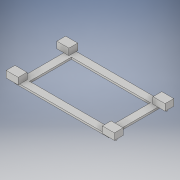
# Autodesk Inventor part: RielesModificado
Saved by Autodesk Inventor 2018 (Build 220112000, 112)
## iProperties
Created: 2021-03-23
Part Number: RielesModificado
Material: Generic
Document SubType Name: Modeling
Designer: Familia
Density: 1 g/cm^3
Appearance: Default
Author: Familia
Autodesk Inventor part; units mm, degrees
ref_plane "YZ Plane" through (0, 0, 0) normal (1, 0, 0) x (0, 1, 0)
ref_plane "XZ Plane" through (0, 0, 0) normal (0, 1, 0) x (-1, 0, 0)
ref_plane "XY Plane" through (0, 0, 0) normal (0, 0, 1) x (1, 0, 0)
sketch "Sketch1" plane through (0, 0, 0) normal (0, 0, 1) x (1, 0, 0)
  line L0 (187.5, -112.5) -> (-187.5, -112.5)
  line L1 (-187.5, -112.5) -> (-187.5, 112.5)
  line L2 (-187.5, 112.5) -> (187.5, 112.5)
  line L3 (187.5, 112.5) -> (187.5, -112.5)
  line L4 (187.5, -112.5) -> (-187.5, 112.5) construction
  line L5 (-187.5, -112.5) -> (187.5, 112.5) construction
  line L6 (157.5, -83.3937) -> (-157.5, -83.3937)
  line L7 (-157.5, -83.3937) -> (-157.5, 83.3937)
  line L8 (-157.5, 83.3937) -> (157.5, 83.3937)
  line L9 (157.5, 83.3937) -> (157.5, -83.3937)
  line L10 (157.5, -83.3937) -> (-157.5, 83.3937) construction
  line L11 (-157.5, -83.3937) -> (157.5, 83.3937) construction
  point P0 (0, 0)
  dimension "d0" = 375
  dimension "d1" = 225
  dimension "d2" = 315
  constraints: 24 end point, 4 midpoint, 4 parallel, 2 horizontal, 2 perpendicular
  measures "d0" distance of L1.end L2.end
  measures "d1" distance of L0.end L1.end
  measures "d2" distance of L7.end L8.end
extrude "Extrusion1" add sketch "Sketch1" along normal blind 7.5
sketch "Sketch2" plane through (0, 0, 7.5) normal (0, 0, 1) x (1, 0, 0)
  line L0 (-157.5, 83.3937) -> (157.5, 83.3937) projected
  line L1 (-167.5, 83.3937) -> (-167.5, 118.3937)
  line L2 (-167.5, 118.3937) -> (-215.5, 118.3937)
  line L3 (-215.5, 118.3937) -> (-215.5, 83.3937)
  line L4 (-215.5, 83.3937) -> (-167.5, 83.3937)
  line L5 (167.5, 83.3937) -> (215.5, 83.3937)
  line L6 (215.5, 83.3937) -> (215.5, 118.3937)
  line L7 (215.5, 118.3937) -> (167.5, 118.3937)
  line L8 (167.5, 118.3937) -> (167.5, 83.3937)
  line L9 (157.5, -83.3937) -> (-157.5, -83.3937) projected
  line L10 (167.5, -83.3937) -> (215.5, -83.3937)
  line L11 (215.5, -83.3937) -> (215.5, -118.3937)
  line L12 (215.5, -118.3937) -> (167.5, -118.3937)
  line L13 (167.5, -118.3937) -> (167.5, -83.3937)
  line L14 (-167.5, -83.3937) -> (-215.5, -83.3937)
  line L15 (-215.5, -83.3937) -> (-215.5, -118.3937)
  line L16 (-215.5, -118.3937) -> (-167.5, -118.3937)
  line L17 (-167.5, -118.3937) -> (-167.5, -83.3937)
  point P0 (0, 0)
  dimension "d5" = 10
  dimension "d6" = 35
  dimension "d7" = 48
  dimension "d8" = 35
  dimension "d9" = 10
  dimension "d10" = 48
  dimension "d11" = 35
  dimension "d12" = 10
  dimension "d13" = 48
  dimension "d14" = 35
  dimension "d15" = 48
  dimension "d16" = 10
  dimension "d17" = 48
  dimension "d18" = 35
  dimension "d19" = 48
  constraints: 32 end point, 8 perpendicular, 1 horizontal, 1 vertical
  measures "d5" distance of L0.start L1.start
  measures "d6" distance of L1.start L1.end
  measures "d7" distance of L1.end L2.end
  measures "d8" distance of L2.end L3.end
  measures "d9" distance of L0.end L5.start
  measures "d10" distance of L5.start L5.end
  measures "d11" distance of L5.end L6.end
  measures "d12" distance of L9.start L10.start
  measures "d13" distance of L10.start L10.end
  measures "d14" distance of L10.end L11.end
  measures "d15" distance of L11.end L12.end
  measures "d16" distance of L9.end L14.start
  measures "d17" distance of L14.start L14.end
  measures "d18" distance of L14.end L15.end
  measures "d19" distance of L15.end L16.end
extrude "Extrusion2" add sketch "Sketch2" along normal blind 26
sketch "Sketch3" plane through (0, 0, 7.5) normal (0, 0, -1) x (-1, 0, 0)
  circle A0 centre (-203.5, 100.8937) radius 4
  line L0 (-187.5, -83.3937) -> (-215.5, -83.3937) projected
  line L1 (167.5, 118.3937) -> (215.5, 118.3937) projected
  line L2 (215.5, 118.3937) -> (215.5, 83.3937) projected
  circle A1 centre (-203.5, -100.8937) radius 4
  circle A2 centre (203.5, -100.8937) radius 4
  circle A3 centre (203.5, 100.8937) radius 4
  point P0 (0, 0)
  point P1 (-215.5, 118.3937)
  point P2 (215.5, -118.3937)
  dimension "d24" = 8
  dimension "d30" = 8
  dimension "d31" = 100.8937
  dimension "d32" = 203.5
  dimension "d33" = 203.5
  dimension "d34" = 100.8937
  dimension "d35" = 100.8937
  dimension "d36" = 203.5
  dimension "d37" = 100.8937
  dimension "d38" = 203.5
  constraints: 4 centre point
  measures "d24" diameter of A0
  measures "d30" diameter of A1
  measures "d31" vertical distance of point (0, 0) A0.centre
  measures "d32" horizontal distance of point (0, 0) A0.centre
  measures "d33" horizontal distance of point (0, 0) A3.centre
  measures "d34" vertical distance of point (0, 0) A3.centre
  measures "d35" vertical distance of point (0, 0) A2.centre
  measures "d36" horizontal distance of point (0, 0) A2.centre
  measures "d37" vertical distance of point (0, 0) A1.centre
  measures "d38" horizontal distance of point (0, 0) A1.centre
extrude "Extrusion3" add sketch "Sketch3" along normal blind 12
body "Solid1"
